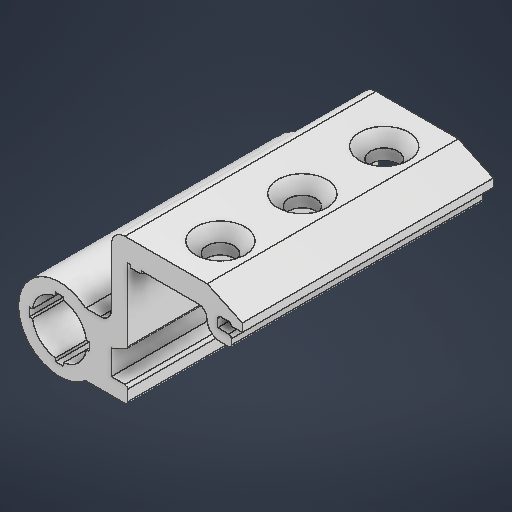
# Autodesk Inventor part: HIN-61 BISAGRA
Saved by Autodesk Inventor 2025 (Build 290162000, 162)
## iProperties
Created: 2026-02-04
Part Number: HIN-61 BISAGRA
Material: Aluminio
Document SubType Name: Modeling
Designer: ROLANDO
Density: 2.7 g/cm^3
Appearance: Satinado
Author: ROLANDO
Autodesk Inventor part; units mm, degrees
ref_plane "YZ Plane" through (0, 0, 0) normal (1, 0, 0) x (0, 1, 0)
ref_plane "XZ Plane" through (0, 0, 0) normal (0, 1, 0) x (-1, 0, 0)
ref_plane "XY Plane" through (0, 0, 0) normal (0, 0, 1) x (1, 0, 0)
sketch "Boceto1" plane through (0, 0, 0) normal (0, 0, 1) x (1, 0, 0)
  arc A0 (4.8153, 5.75) -> (4.8153, -5.75) centre (0, 0) ccw
  line L0 (0, 12.1119) -> (0, -11.4197) construction
  line L1 (-11.1817, 0) -> (12.1806, 0) construction
  line L2 (4.9434, 0.75) -> (5.5, 0.75)
  line L3 (4.9434, -0.75) -> (5.5, -0.75)
  line L4 (5.5, -0.75) -> (5.5, 0.75)
  line L5 (-0.75, 4.9434) -> (-0.75, 5.5)
  line L6 (0.75, 5.5) -> (-0.75, 5.5)
  line L7 (0.75, 4.9434) -> (0.75, 5.5)
  line L8 (-4.9434, -0.75) -> (-5.5, -0.75)
  line L9 (-5.5, 0.75) -> (-5.5, -0.75)
  line L10 (-4.9434, 0.75) -> (-5.5, 0.75)
  line L11 (0.75, -4.9434) -> (0.75, -5.5)
  line L12 (-0.75, -5.5) -> (0.75, -5.5)
  line L13 (-0.75, -4.9434) -> (-0.75, -5.5)
  arc A1 (-0.75, 4.9434) -> (-4.9434, 0.75) centre (0, 0) ccw
  arc A2 (-4.9434, -0.75) -> (-0.75, -4.9434) centre (0, 0) ccw
  arc A3 (0.75, -4.9434) -> (4.9434, -0.75) centre (0, 0) ccw
  arc A4 (4.9434, 0.75) -> (0.75, 4.9434) centre (0, 0) ccw
  circle A5 centre (0, 0) radius 5 construction
  line L14 (-11.772, 7.5) -> (14.517, 7.5) construction
  line L15 (-11.772, -7.5) -> (14.517, -7.5) construction
  line L16 (4.8153, 5.75) -> (7.5, 5.75)
  line L17 (9.5, 7.75) -> (9.5, 18.25)
  line L18 (12, 20.75) -> (27.0665, 20.75)
  line L19 (31.5, 16.25) -> (31.5, 16.25)
  line L20 (31, 16.75) -> (29.5, 16.75)
  line L21 (29, 16.25) -> (29, 14.75)
  line L22 (29, 14.75) -> (31, 14.75)
  line L23 (31.5, 14.25) -> (31.5, 13.25)
  line L24 (31, 12.75) -> (29.4417, 12.75)
  line L25 (27, 15.1917) -> (27, 15.25)
  line L26 (25.5, 16.75) -> (15, 16.75)
  line L27 (15, 16.75) -> (15, 16.25)
  line L28 (15, 16.25) -> (13, 16.25)
  line L29 (13, 16.25) -> (13, 16.75)
  line L30 (13, 16.75) -> (12.5, 16.75)
  line L31 (12.5, 16.75) -> (12.5, 3.4675)
  line L32 (12.2113, 3.0143) -> (9.5, 1.75)
  line L33 (9.5, 1.75) -> (9.5, -2.75)
  line L34 (9.5, -2.75) -> (12, -2.75)
  line L35 (12.5, -3.25) -> (12.5, -5.25)
  line L36 (12, -5.75) -> (4.8153, -5.75)
  line L37 (33.5, 16.25) -> (33.5, 17.75)
  line L38 (31.5, 16.25) -> (33.5, 16.25)
  arc A6 (31, 12.75) -> (31.5, 13.25) centre (31, 13.25) ccw
  arc A7 (31.5, 14.25) -> (31, 14.75) centre (31, 14.25) ccw
  arc A8 (31.5, 16.25) -> (31, 16.75) centre (31, 16.25) ccw
  arc A9 (29.5, 16.75) -> (29, 16.25) centre (29.5, 16.25) ccw
  arc A10 (27, 15.25) -> (25.5, 16.75) centre (25.5, 15.25) ccw
  arc A11 (27, 15.1917) -> (29.4417, 12.75) centre (29.4417, 15.1917) ccw
  arc A12 (12, 20.75) -> (9.5, 18.25) centre (12, 18.25) ccw
  arc A13 (12.2113, 3.0143) -> (12.5, 3.4675) centre (12, 3.4675) ccw
  arc A14 (12.5, -3.25) -> (12, -2.75) centre (12, -3.25) ccw
  arc A15 (12, -5.75) -> (12.5, -5.25) centre (12, -5.25) ccw
  arc A16 (7.5, 5.75) -> (9.5, 7.75) centre (7.5, 7.75) ccw
  line L39 (33.5, 17.75) -> (27.0665, 20.75)
  point P0 (31.5, 14.75)
  point P1 (31.5, 12.75)
  point P2 (27, 12.75)
  point P3 (27, 16.75)
  point P4 (12.5, -2.75)
  point P5 (12.5, -5.75)
  point P6 (-7.5, 0)
  point P7 (5.5, 0)
  dimension "d0" = 15
  dimension "d4" = 0.75
  dimension "d6" = 1.5
  dimension "d11" = 360
  dimension "d13" = 10
  dimension "d14" = 0.5
  dimension "d15" = 5
  dimension "d16" = 1.75
  dimension "d17" = 1.75
  dimension "d18" = 11.5
  dimension "d20" = 3
  dimension "d21" = 3
  dimension "d22" = 3
  dimension "d23" = 4
  dimension "d24" = 115
  dimension "d26" = 19
  dimension "d27" = 15
  dimension "d28" = 0.5
  dimension "d30" = 0.5
  dimension "d31" = 8
  dimension "d33" = 0.5
  dimension "d36" = 2
  dimension "d41" = 65
  dimension "d43" = 0.5
  dimension "d44" = 0.5
  dimension "d45" = 1.5
  dimension "d47" = 2.5
  dimension "d48" = 0.5
  dimension "d49" = 2
  dimension "d88" = 20
  dimension "d89" = 4
  dimension "d92" = 28.25
  dimension "d93" = 2
  dimension "d94" = 2
  dimension "d95" = 14.5
  dimension "d96" = 2.4417
  dimension "d98" = 155
  dimension "d99" = 2
  dimension "d101" = 1.5
  dimension "d102" = 2.5
  dimension "d103" = 24
  constraints: 80 end point, 33 point on circle, 24 tangent, 22 point on line, 17 centre point, 14 perpendicular, 6 horizontal, 4 equal radius, 3 coincident, 3 vertical, 1 collinear, 1 midpoint, 29 other
  measures "d0" diameter of A0
  measures "d4" distance between parallel lines of L1 L3
  measures "d6" distance between parallel lines of L3 L2
  measures "d13" diameter of A5
  measures "d14" distance edge to line of A5 L6
  measures "d15" radius of A4
  measures "d16" distance between parallel lines of L14 L16
  measures "d17" distance between parallel lines of L15 L36
  measures "d18" distance between parallel lines of L36 L16
  measures "d20" distance between parallel lines of L36 L34
  measures "d21" distance between parallel lines of L33 L35
  measures "d22" distance between parallel lines of L17 L31
  measures "d23" distance between parallel lines of L18 L26
  measures "d24" angle of L31 L32
  measures "d26" distance from line of L18 L32.end
  measures "d27" distance between parallel lines of L18 L16
  measures "d28" distance between parallel lines of L31 L29
  measures "d30" distance of L26.end L27.end
  measures "d31" distance between parallel lines of L24 L18
  measures "d33" distance between parallel lines of L38 L20
  measures "d36" distance between parallel lines of L25 L21
  measures "d41" angle of L17 L32
  measures "d43" radius of A6
  measures "d44" radius of A8
  measures "d45" radius of A10
  measures "d47" radius of A12
  measures "d48" radius of A13
  measures "d49" radius of A16
  measures "d88" distance from line of point (-7.5, 0) L31
  measures "d89" distance from line of point (5.5, 0) L33
  measures "d92" distance between parallel lines of L18 L15
  measures "d93" distance of L27.end L28.end
  measures "d94" distance between parallel lines of L22 L24
  measures "d95" distance between parallel lines of L31 L25
  measures "d96" radius of A11
  measures "d98" angle of L18 L39
  measures "d99" distance of L19.start L37.start
  measures "d101" distance of L37.start L37.end
  measures "d102" distance from line of L21 L19.start
  measures "d103" distance between parallel lines of L37 L17
extrude "Extrusión1" add sketch "Boceto1" against normal blind 46
sketch "Boceto2" plane through (12, 20.75, 0) normal (0, 1, 0) x (1, 0, 0)
  line L0 (9.4815, 49.0857) -> (9.4815, -3.1706) construction
  line L1 (20.8474, 23) -> (-1.8844, 23) construction
  line L2 (0, 0) -> (0, 46) construction
  line L3 (15.0665, 0) -> (0, 0) construction
  line L4 (0, 46) -> (15.0665, 46) construction
  circle A0 centre (9.4815, 23) radius 2.5
  circle A1 centre (9.4815, 23) radius 4.5
  circle A2 centre (9.4815, 8) radius 2.5
  circle A3 centre (9.4815, 8) radius 4.5
  circle A4 centre (9.4815, 38) radius 2.5
  circle A5 centre (9.4815, 38) radius 4.5
  line L5 (15.0665, 0) -> (15.0665, 46) projected
  point P0 (-12, 0)
  dimension "d67" = 23
  dimension "d68" = 23
  dimension "d69" = 5
  dimension "d70" = 9
  dimension "d72" = 2
  dimension "d75" = 15
  dimension "d104" = 5.585
  constraints: 6 centre point, 4 end point, 3 coincident, 2 vertical, 1 horizontal, 1 midpoint, 1 point on line, 8 other
  measures "d67" distance between parallel lines of L3 L1
  measures "d68" distance between parallel lines of L4 L1
  measures "d69" diameter of A0
  measures "d70" diameter of A1
  measures "d72" radial gap between concentric circles of A1 A0
  measures "d75" distance of A0.centre A2.centre
  measures "d104" distance between parallel lines of L5 L0
hole "Agujero1" at (21.4815, 20.75, -38) at (21.4815, 20.75, -23) at (21.4815, 20.75, -8) direction (0, -1, 0) diameter 5 end through all countersink diameter 9 countersink angle 90
